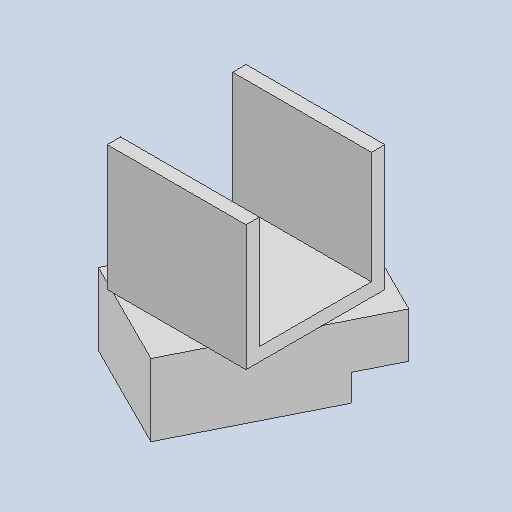
# Autodesk Inventor part: camera_case2
Saved by Autodesk Inventor 2025.2 (Build 292293000, 293)
## iProperties
Created: 2024-02-22
Part Number: camera_case2
Material: 일반
Document SubType Name: Modeling
Designer: ps737
Density: 1 g/cm^3
Appearance: 기본값
Author: ps737
Autodesk Inventor part; units mm, degrees
ref_plane "YZ Plane" through (0, 0, 0) normal (1, 0, 0) x (0, 1, 0)
ref_plane "XZ Plane" through (0, 0, 0) normal (0, 1, 0) x (-1, 0, 0)
ref_plane "XY Plane" through (0, 0, 0) normal (0, 0, 1) x (1, 0, 0)
sketch "스케치1" plane through (0, 0, 0) normal (0, 1, 0) x (-1, 0, 0)
  line L0 (0, 0) -> (-52, 0)
  line L1 (-52, 0) -> (-52, -52)
  line L2 (-52, -52) -> (0, -52)
  line L3 (0, -52) -> (0, 0)
  line L4 (-52, -5) -> (0, -5)
  line L5 (0, -47) -> (-52, -47)
  dimension "d0" = 52
  dimension "d1" = 52
  dimension "d2" = 5
  dimension "d7" = 5
  constraints: 12 end point, 4 point on line, 3 parallel, 1 coincident, 1 horizontal, 1 perpendicular
  measures "d0" distance of L2.end L1.end
  measures "d1" distance of L1.end L0.end
  measures "d2" distance between parallel lines of L0 L4
  measures "d7" distance between parallel lines of L2 L5
extrude "돌출1" add sketch "스케치1" along normal blind 5 contours L3 L5 L1 L4
extrude "돌출2" add sketch "스케치1" along normal blind 47 contours L3 L4 L1 L0 | L3 L2 L1 L5
sketch "스케치2" plane through (0, 0, 0) normal (0, -1, 0) x (1, 0, 0)
  line L0 (52, -52) -> (0, -52) projected
  line L1 (52, -52) -> (52, -32)
  line L2 (52, 0) -> (52, -52) projected
  line L3 (52, -52) -> (42, -52)
  line L4 (42, -52) -> (52, -32)
  line L5 (42, -52) -> (32.1613, -71.6774)
  line L6 (32.1613, -71.6774) -> (64.3607, -7.2786)
  line L7 (64.3607, -7.2786) -> (21.4282, 14.1876)
  line L8 (21.4282, 14.1876) -> (-10.7712, -50.2111)
  line L9 (-10.7712, -50.2111) -> (32.1613, -71.6774)
  line L10 (-5.4046, -48.4223) -> (23.217, 8.821)
  line L11 (23.217, 8.821) -> (58.9941, -9.0675)
  line L12 (58.9941, -9.0675) -> (30.3724, -66.3108)
  line L13 (33.9502, -68.0997) -> (-5.4046, -48.4223)
  line L14 (60.783, -5.4898) -> (55.8636, -15.3285)
  line L15 (55.8636, -15.3285) -> (59.4413, -17.1173)
  point P0 (0, 0)
  dimension "d0" = 52
  dimension "d1" = 52
  dimension "d2" = 5
  dimension "d7" = 5
  dimension "d8" = 20
  dimension "d9" = 10
  dimension "d10" = 22
  dimension "d11" = 72
  dimension "d12" = 48
  dimension "d13" = 4
  dimension "d14" = 11
  dimension "d24" = 26.565
  dimension "d25" = 72
  constraints: 28 end point, 9 point on line, 7 perpendicular, 2 other
  measures "d8" distance of L0.start L1.end
  measures "d9" distance of L0.start L3.end
  measures "d10" distance of L3.end L5.end
  measures "d11" distance of L5.end L6.end
  measures "d12" distance of L6.end L7.end
  measures "d13" distance between parallel lines of L8 L10
  measures "d14" distance of L14.start L14.end
  measures "d24" angle of L2 L4
  measures "d25" distance between parallel lines of L7 L9
extrude "돌출3" add sketch "스케치2" along normal blind 4 contours L5 L13 L12 L0 | L0 L12 L2 L4 | L2 L12 L15 L6 | L12 L13 L0 | L0 L13 L10 L11 L2 L12 | L2 L11 L12
extrude "돌출4" add sketch "스케치2" along normal blind 27 contours L5 L9 L8 L7 L2 L11 L10 L13 | L2 L7 L14 L11
sketch "스케치3" plane through (58.9941, -27, -9.0675) normal (-0.4472136, 0, -0.8944272) x (-0.8944272, 0, 0.4472136)
  line L0 (0, 23) -> (0, 0) projected
  line L1 (0, 0) -> (0, 4)
  line L2 (0, 4) -> (40, 4)
  line L3 (40, 23) -> (40, 0) projected
  line L4 (40, 0) -> (0, 0) projected
  point P0 (56.821, 27)
  dimension "d19" = 4
  constraints: 4 end point, 2 point on line, 1 perpendicular
  measures "d19" distance of L0.end L1.end
extrude "돌출5" add sketch "스케치3" along normal blind 52
sketch "스케치4" plane through (0, -27, 0) normal (0, -1, 0) x (1, 0, 0)
  line L0 (32.1613, -71.6774) -> (33.9502, -68.0997) projected
  line L1 (33.9502, -68.0997) -> (-5.4046, -48.4223) projected
  line L2 (-5.4046, -48.4223) -> (-0.0381, -37.6892) projected
  line L3 (35.739, -55.5777) -> (-0.0381, -37.6892) projected
  line L4 (60.783, -5.4898) -> (35.739, -55.5777) projected
  line L5 (60.783, -5.4898) -> (21.4282, 14.1876) projected
  line L6 (21.4282, 14.1876) -> (-10.7712, -50.2111) projected
  line L7 (-10.7712, -50.2111) -> (32.1613, -71.6774) projected
  line L8 (-0.0381, -37.6892) -> (-3.6158, -35.9003)
  line L9 (32.1613, -71.6774) -> (42, -52) projected
  line L10 (33.9502, -68.0997) -> (32.1613, -71.6774)
  line L11 (32.1613, -71.6774) -> (-10.7712, -50.2111)
  line L12 (-3.6158, -35.9003) -> (-0.0381, -37.6892)
  point P0 (0, 0)
  constraints: 8 end point, 3 collinear, 1 perpendicular, 1 point on line
extrude "돌출6" cut sketch "스케치4" against normal blind 10 contours L7 L6 L8 L2 L1 L0
mirror "미러1" about plane through (0, 0, 0) normal (1, 0, 0) remove original yes
